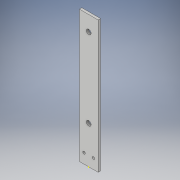
# Autodesk Inventor part: Main Support
Saved by Autodesk Inventor 2018 (Build 220112000, 112)
## iProperties
Created: 2017-04-14
Part Number: Main Support
Material: Generic
Document SubType Name: Modeling
Designer: Administrator
Density: 1 g/cm^3
Appearance: Default
Author: Administrator
Autodesk Inventor part; units mm, degrees
ref_plane "YZ Plane" through (0, 0, 0) normal (1, 0, 0) x (0, 1, 0)
ref_plane "XZ Plane" through (0, 0, 0) normal (0, 1, 0) x (-1, 0, 0)
ref_plane "XY Plane" through (0, 0, 0) normal (0, 0, 1) x (1, 0, 0)
sketch "Sketch1" plane through (0, 0, 0) normal (0, 0, 1) x (1, 0, 0)
  line L0 (-25, 0) -> (25, 0)
  line L1 (25, 0) -> (25, 350)
  line L2 (25, 350) -> (-25, 350)
  line L3 (-25, 350) -> (-25, 0)
  circle A0 centre (0, 100.214) radius 6.35
  circle A1 centre (0, 310) radius 6.35
  circle A2 centre (-12.5, 26.5) radius 3.25
  circle A3 centre (12.5, 26.5) radius 3.25
  point P0 (0, 0)
  dimension "d0" = 50
  dimension "d1" = 350
  dimension "d2" = 12.7
  dimension "d3" = 12.7
  dimension "d4" = 6.5
  dimension "d5" = 6.5
  constraints: 8 end point, 4 centre point, 2 parallel, 1 horizontal, 1 perpendicular
  measures "d0" distance of L2.end L1.end
  measures "d1" distance of L1.end L0.end
  measures "d2" diameter of A0
  measures "d3" diameter of A1
  measures "d4" diameter of A2
  measures "d5" diameter of A3
extrude "Extrusion1" add sketch "Sketch1" along normal blind 6.5
sketch "Sketch2" plane through (0, 0, 6.5) normal (0, 0, 1) x (1, 0, 0)
  point P0 (0, 0)
body "Solid1"
